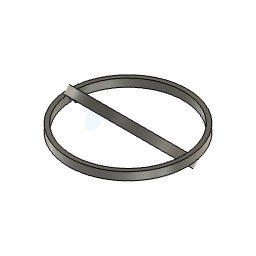
Villagers_E_Waste_Sorter_autocadmode v1 (Autodesk Fusion 360 archive; units mm, degrees)
design "final drop mech"
Autodesk Fusion 360 part; units mm, degrees
sketch "Sketch1" plane through (0, 0, 0) normal (0, 0, 1) x (1, 0, 0)
  circle A0 centre (0, 0) radius 75
  dimension "d1" = 150
  constraint coincident A0.centre origin
  measures "d1" diameter of A0
extrude "Extrude1" add sketch "Sketch1" along normal blind 10 makes body 1
sketch "Sketch2" plane through (0, 0, 10) normal (0, 0, 1) x (-1, 0, 0)
  circle A0 centre (0, 0) radius 75
  circle A1 centre (0, 0) radius 70
  dimension "d4" = 140
  constraint coincident A0.centre A1.centre
  measures "d4" diameter of A1
extrude "Extrude2" cut sketch "Sketch2" against normal blind 20 contours A1 bodies 1
sketch "Sketch3" plane through (0, 0, 0) normal (1, 0, 0) x (0, 1, 0)
  circle A0 centre (0, 40) radius 4
  dimension "d7" = 8
  measures "d7" diameter of A0
extrude "Extrude3" add sketch "Sketch3" along normal blind 8 separate body makes body 2
copy_body "CopyPasteBodies1" bodies 2 makes body 3
move_body "Move4" bodies 3 to x (1, 0, 0) y (0, 1, 0) z (0, 0, 1) at (0, 0, 0)
move_body "Move5" bodies 3 to x (1, 0, 0) y (0, 1, 0) z (0, 0, 1) at (64, 0, -35)
move_body "Move6" bodies 2 to x (1, 0, 0) y (0, 1, 0) z (0, 0, 1) at (-8, 0, -30)
move_body "Move7" bodies 2 to x (1, 0, 0) y (0, 1, 0) z (0, 0, 1) at (-62, 0, -5)
move_body "Move8" bodies 2 to x (1, 0, 0) y (0, 1, 0) z (0, 0, 1) at (-2, 0, 0)
sketch "Sketch4" plane through (-64, 0, 0) normal (1, 0, 0) x (0, 1, 0)
  circle A0 centre (0, 5) radius 4
sketch "Sketch5" plane through (0, 0, 0) normal (0, 0, 1) x (1, 0, 0)
  circle A0 centre (0, 0) radius 66.9423
  constraint coincident A0.centre origin
extrude "Extrude4" add sketch "Sketch5" against normal blind 10 separate body makes body 4
sketch "Sketch6" plane through (0, 0, 0) normal (0, 0, 1) x (1, 0, 0)
move_body "Move9" bodies 4 to x (1, 0, 0) y (0, 0.707107, -0.707107) z (0, 0.707107, 0.707107) at (0, 17.2128, 86.9108)
move_body "Move10" bodies 4 to x (1, 0, 0) y (0, 1, 0) z (0, 0, 1) at (15.5398, -10.1268, -3.5597)
sketch "Sketch7" plane through (0, 38.1475, 38.1475) normal (0, -0.707107, -0.707107) x (1, 0, 0)
sketch "Sketch8" plane through (0, 38.1475, 38.1475) normal (0, -0.707107, -0.707107) x (1, 0, 0)
combine "Combine2" operation add target body 3 tool bodies 1 2
move_body "Move11" bodies 4 to x (1, 0, 0) y (0, 1, 0) z (0, 0, 1) at (-15, 0, -75)
scale "Scale1" factor 0.333333 about (-75, 0, 10) bodies 4 3
move_body "Move1" [suppressed]
move_body "Move2" [suppressed]
move_body "Move3" [suppressed]
combine "Combine1" [suppressed]
equation "d12 = 1 / 3"
